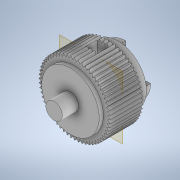
# Autodesk Inventor part: PotAttachmentB10L
Saved by Autodesk Inventor 2022 (Build 260153000, 153)
## iProperties
Created: 2021-10-23
Part Number: PotAttachmentB10L
Material: Generic
Document SubType Name: Modeling
Designer: teh18
Density: 1 g/cm^3
Appearance: Default
Author: teh18
Autodesk Inventor part; units mm, degrees
ref_plane "YZ Plane" through (0, 0, 0) normal (1, 0, 0) x (0, 1, 0)
ref_plane "XZ Plane" through (0, 0, 0) normal (0, 1, 0) x (-1, 0, 0)
ref_plane "XY Plane" through (0, 0, 0) normal (0, 0, 1) x (1, 0, 0)
sketch "Sketch1" plane through (0, 0, 0) normal (0, 0, 1) x (1, 0, 0)
  arc A0 (-0.1225, 6.9989) -> (-6, 3.6056) centre (0, 0) ccw projected
  circle A1 centre (0, 0) radius 7
  line L0 (0, -12) -> (0, -10) projected
  arc A2 (0, -10) -> (10, 0) centre (0, 0) ccw projected
  line L1 (10, 0) -> (12, 0) projected
  arc A3 (0, -12) -> (12, 0) centre (0, 0) ccw projected
  line L2 (0, 12) -> (0, 10) projected
  arc A4 (0, 10) -> (-10, 0) centre (0, 0) ccw projected
  line L3 (-10, 0) -> (-12, 0) projected
  arc A5 (0, 12) -> (-12, 0) centre (0, 0) ccw projected
  arc A6 (4.4269, -19.95) -> (6.1412, -19.4907) centre (5.1647, -19.275) ccw projected
  arc A7 (13.8088, -15.0638) -> (6.1412, -19.4907) centre (12, -20.7846) ccw projected
  arc A8 (13.8088, -15.0638) -> (15.0638, -13.8088) centre (14.1103, -14.1103) ccw projected
  arc A9 (19.4907, -6.1412) -> (15.0638, -13.8088) centre (20.7846, -12) ccw projected
  arc A10 (19.4907, -6.1412) -> (19.95, -4.4269) centre (19.275, -5.1647) ccw projected
  arc A11 (27.8571, 4.5959) -> (19.95, -4.4269) centre (24, 0) ccw projected
  arc A12 (27.8571, 4.5959) -> (29.4828, 5.5468) centre (28.5, 5.3619) ccw projected
  arc A13 (29.4828, 5.5468) -> (27.5804, 11.8035) centre (0, 0) ccw projected
  line L4 (27.5804, 11.8035) -> (33.0964, 14.1643) projected
  arc A14 (33.0964, 14.1643) -> (26.445, 24.4267) centre (0, 0) ccw projected
  line L5 (26.445, 24.4267) -> (22.0375, 20.3556) projected
  arc A15 (22.0375, 20.3556) -> (-20.3556, 22.0375) centre (0, 0) ccw projected
  line L6 (-20.3556, 22.0375) -> (-16.2845, 17.63) projected
  arc A16 (-16.2845, 17.63) -> (-5.9529, -23.25) centre (0, 0) ccw projected
  arc A17 (4.4269, -19.95) -> (-5.9529, -23.25) centre (0, -24) ccw projected
  arc A18 (-1, 6.9282) -> (-6.9282, 1) centre (0, 0) ccw projected
  line L7 (-1, 6.9282) -> (-1, 1) projected
  line L8 (-1, 1) -> (-6.9282, 1) projected
  line L9 (-6.9282, -1) -> (-1, -1) projected
  line L10 (-1, -1) -> (-1, -6.9282) projected
  arc A19 (-6.9282, -1) -> (-1, -6.9282) centre (0, 0) ccw projected
  line L11 (1, -6.9282) -> (1, -1) projected
  line L12 (1, -1) -> (6.9282, -1) projected
  arc A20 (1, -6.9282) -> (6.9282, -1) centre (0, 0) ccw projected
  line L13 (6.9282, 1) -> (1, 1) projected
  line L14 (1, 1) -> (1, 6.9282) projected
  arc A21 (6.9282, 1) -> (1, 6.9282) centre (0, 0) ccw projected
  circle A22 centre (0, 0) radius 14
  point P0 (0, 0)
  point P1 (-6, 3.6056)
  point P2 (-0.1225, 6.9989)
  dimension "d2" = 28
  constraints: 1 centre point, 1 coincident, 2 other
  measures "d2" diameter of A22
extrude "Extrusion1" add sketch "Sketch1" along normal blind 23 contours L0 A2 L1 A3 | L2 A4 L3 A5 | A22
sketch "Sketch2" plane through (0, 0, 0) normal (0, 0, -1) x (-1, 0, 0)
  line L0 (0, -12) -> (0, -10) projected
  arc A0 (-10, 0) -> (0, -10) centre (0, 0) ccw projected
  line L1 (-10, 0) -> (-12, 0) projected
  arc A1 (-12, 0) -> (0, -12) centre (0, 0) ccw projected
  line L2 (0, 12) -> (0, 10) projected
  arc A2 (10, 0) -> (0, 10) centre (0, 0) ccw projected
  line L3 (10, 0) -> (12, 0) projected
  arc A3 (12, 0) -> (0, 12) centre (0, 0) ccw projected
  arc A4 (-6.1412, -19.4907) -> (-4.4269, -19.95) centre (-5.1647, -19.275) ccw projected
  arc A5 (-6.1412, -19.4907) -> (-13.8088, -15.0638) centre (-12, -20.7846) ccw projected
  arc A6 (-15.0638, -13.8088) -> (-13.8088, -15.0638) centre (-14.1103, -14.1103) ccw projected
  arc A7 (-15.0638, -13.8088) -> (-19.4907, -6.1412) centre (-20.7846, -12) ccw projected
  arc A8 (-19.95, -4.4269) -> (-19.4907, -6.1412) centre (-19.275, -5.1647) ccw projected
  arc A9 (-19.95, -4.4269) -> (-27.8571, 4.5959) centre (-24, 0) ccw projected
  arc A10 (-29.4828, 5.5468) -> (-27.8571, 4.5959) centre (-28.5, 5.3619) ccw projected
  arc A11 (-27.5804, 11.8035) -> (-29.4828, 5.5468) centre (0, 0) ccw projected
  line L4 (-27.5804, 11.8035) -> (-33.0964, 14.1643) projected
  arc A12 (-26.445, 24.4267) -> (-33.0964, 14.1643) centre (0, 0) ccw projected
  line L5 (-26.445, 24.4267) -> (-22.0375, 20.3556) projected
  arc A13 (20.3556, 22.0375) -> (-22.0375, 20.3556) centre (0, 0) ccw projected
  line L6 (20.3556, 22.0375) -> (16.2845, 17.63) projected
  arc A14 (5.9529, -23.25) -> (16.2845, 17.63) centre (0, 0) ccw projected
  arc A15 (5.9529, -23.25) -> (-4.4269, -19.95) centre (0, -24) ccw projected
  arc A16 (6.9282, 1) -> (1, 6.9282) centre (0, 0) ccw projected
  line L7 (1, 6.9282) -> (1, 1) projected
  line L8 (1, 1) -> (6.9282, 1) projected
  line L9 (6.9282, -1) -> (1, -1) projected
  line L10 (1, -1) -> (1, -6.9282) projected
  arc A17 (1, -6.9282) -> (6.9282, -1) centre (0, 0) ccw projected
  line L11 (-1, -6.9282) -> (-1, -1) projected
  line L12 (-1, -1) -> (-6.9282, -1) projected
  arc A18 (-6.9282, -1) -> (-1, -6.9282) centre (0, 0) ccw projected
  line L13 (-6.9282, 1) -> (-1, 1) projected
  line L14 (-1, 1) -> (-1, 6.9282) projected
  arc A19 (-1, 6.9282) -> (-6.9282, 1) centre (0, 0) ccw projected
  point P0 (0, 0)
extrude "Extrusion2" add sketch "Sketch2" along normal blind 4 contours A1 L1 A0 L0 | A3 L3 A2 L2
ref_plane "Work Plane1" through (0, 0, 13) normal (0, 0, 1) x (1, 0, 0)
sketch "Sketch4" plane through (0, 0, 13) normal (0, 0, 1) x (1, 0, 0)
  circle A0 centre (0, 0) radius 3
  circle A1 centre (0, 0) radius 7 projected
  dimension "d10" = 6
  constraints: 1 centre point, 1 coincident
  measures "d10" diameter of A0
extrude "Extrusion4" add sketch "Sketch4" along normal up to surface (10 mm away) contours A0 | A1
sketch "Sketch6" plane through (0, 0, 23) normal (0, 0, 1) x (1, 0, 0)
  circle A0 centre (0, 0) radius 4
  dimension "d25" = 8
  constraints: 1 centre point, 1 coincident
  measures "d25" diameter of A0
extrude "Extrusion6" add sketch "Sketch6" along normal blind 8
sketch "Sketch7" plane through (0, 0, 13) normal (0, 0, 1) x (1, 0, 0)
  circle A0 centre (0, 0) radius 14 projected
  line L0 (0, 17.4641) -> (3, 12.2679)
  line L1 (3, 12.2679) -> (-3, 12.2679)
  line L2 (-3, 12.2679) -> (0, 17.4641)
  line L3 (-1.8255, 17.3684) -> (1.7012, 12.5143)
  line L4 (-4.2659, 11.8872) -> (-1.8255, 17.3684)
  line L5 (1.7012, 12.5143) -> (-4.2659, 11.8872)
  line L6 (-3.631, 17.0825) -> (0.3838, 12.6236)
  line L7 (-5.4851, 11.3761) -> (-3.631, 17.0825)
  line L8 (0.3838, 12.6236) -> (-5.4851, 11.3761)
  line L9 (-5.3967, 16.6093) -> (-0.9378, 12.5946)
  line L10 (-6.6442, 10.7405) -> (-5.3967, 16.6093)
  line L11 (-0.9378, 12.5946) -> (-6.6442, 10.7405)
  line L12 (-7.1033, 15.9543) -> (-2.2492, 12.4275)
  line L13 (-7.7305, 9.9871) -> (-7.1033, 15.9543)
  line L14 (-2.2492, 12.4275) -> (-7.7305, 9.9871)
  line L15 (-8.7321, 15.1244) -> (-3.5359, 12.1244)
  line L16 (-8.7321, 9.1244) -> (-8.7321, 15.1244)
  line L17 (-3.5359, 12.1244) -> (-8.7321, 9.1244)
  line L18 (-10.2651, 14.1288) -> (-4.7839, 11.6883)
  line L19 (-9.638, 8.1616) -> (-10.2651, 14.1288)
  line L20 (-4.7839, 11.6883) -> (-9.638, 8.1616)
  line L21 (-11.6858, 12.9784) -> (-5.9794, 11.1243)
  line L22 (-10.4383, 7.1095) -> (-11.6858, 12.9784)
  line L23 (-5.9794, 11.1243) -> (-10.4383, 7.1095)
  line L24 (-12.9784, 11.6858) -> (-7.1095, 10.4383)
  line L25 (-11.1243, 5.9794) -> (-12.9784, 11.6858)
  line L26 (-7.1095, 10.4383) -> (-11.1243, 5.9794)
  line L27 (-14.1288, 10.2651) -> (-8.1616, 9.638)
  line L28 (-11.6883, 4.7839) -> (-14.1288, 10.2651)
  line L29 (-8.1616, 9.638) -> (-11.6883, 4.7839)
  line L30 (-15.1244, 8.7321) -> (-9.1244, 8.7321)
  line L31 (-12.1244, 3.5359) -> (-15.1244, 8.7321)
  line L32 (-9.1244, 8.7321) -> (-12.1244, 3.5359)
  line L33 (-15.9543, 7.1033) -> (-9.9871, 7.7305)
  line L34 (-12.4275, 2.2492) -> (-15.9543, 7.1033)
  line L35 (-9.9871, 7.7305) -> (-12.4275, 2.2492)
  line L36 (-16.6093, 5.3967) -> (-10.7405, 6.6442)
  line L37 (-12.5946, 0.9378) -> (-16.6093, 5.3967)
  line L38 (-10.7405, 6.6442) -> (-12.5946, 0.9378)
  line L39 (-17.0825, 3.631) -> (-11.3761, 5.4851)
  line L40 (-12.6236, -0.3838) -> (-17.0825, 3.631)
  line L41 (-11.3761, 5.4851) -> (-12.6236, -0.3838)
  line L42 (-17.3684, 1.8255) -> (-11.8872, 4.2659)
  line L43 (-12.5143, -1.7012) -> (-17.3684, 1.8255)
  line L44 (-11.8872, 4.2659) -> (-12.5143, -1.7012)
  line L45 (-17.4641, 0) -> (-12.2679, 3)
  line L46 (-12.2679, -3) -> (-17.4641, 0)
  line L47 (-12.2679, 3) -> (-12.2679, -3)
  line L48 (-17.3684, -1.8255) -> (-12.5143, 1.7012)
  line L49 (-11.8872, -4.2659) -> (-17.3684, -1.8255)
  line L50 (-12.5143, 1.7012) -> (-11.8872, -4.2659)
  line L51 (-17.0825, -3.631) -> (-12.6236, 0.3838)
  line L52 (-11.3761, -5.4851) -> (-17.0825, -3.631)
  line L53 (-12.6236, 0.3838) -> (-11.3761, -5.4851)
  line L54 (-16.6093, -5.3967) -> (-12.5946, -0.9378)
  line L55 (-10.7405, -6.6442) -> (-16.6093, -5.3967)
  line L56 (-12.5946, -0.9378) -> (-10.7405, -6.6442)
  line L57 (-15.9543, -7.1033) -> (-12.4275, -2.2492)
  line L58 (-9.9871, -7.7305) -> (-15.9543, -7.1033)
  line L59 (-12.4275, -2.2492) -> (-9.9871, -7.7305)
  line L60 (-15.1244, -8.7321) -> (-12.1244, -3.5359)
  line L61 (-9.1244, -8.7321) -> (-15.1244, -8.7321)
  line L62 (-12.1244, -3.5359) -> (-9.1244, -8.7321)
  line L63 (-14.1288, -10.2651) -> (-11.6883, -4.7839)
  line L64 (-8.1616, -9.638) -> (-14.1288, -10.2651)
  line L65 (-11.6883, -4.7839) -> (-8.1616, -9.638)
  line L66 (-12.9784, -11.6858) -> (-11.1243, -5.9794)
  line L67 (-7.1095, -10.4383) -> (-12.9784, -11.6858)
  line L68 (-11.1243, -5.9794) -> (-7.1095, -10.4383)
  line L69 (-11.6858, -12.9784) -> (-10.4383, -7.1095)
  line L70 (-5.9794, -11.1243) -> (-11.6858, -12.9784)
  line L71 (-10.4383, -7.1095) -> (-5.9794, -11.1243)
  line L72 (-10.2651, -14.1288) -> (-9.638, -8.1616)
  line L73 (-4.7839, -11.6883) -> (-10.2651, -14.1288)
  line L74 (-9.638, -8.1616) -> (-4.7839, -11.6883)
  line L75 (-8.7321, -15.1244) -> (-8.7321, -9.1244)
  line L76 (-3.5359, -12.1244) -> (-8.7321, -15.1244)
  line L77 (-8.7321, -9.1244) -> (-3.5359, -12.1244)
  line L78 (-7.1033, -15.9543) -> (-7.7305, -9.9871)
  line L79 (-2.2492, -12.4275) -> (-7.1033, -15.9543)
  line L80 (-7.7305, -9.9871) -> (-2.2492, -12.4275)
  line L81 (-5.3967, -16.6093) -> (-6.6442, -10.7405)
  line L82 (-0.9378, -12.5946) -> (-5.3967, -16.6093)
  line L83 (-6.6442, -10.7405) -> (-0.9378, -12.5946)
  line L84 (-3.631, -17.0825) -> (-5.4851, -11.3761)
  line L85 (0.3838, -12.6236) -> (-3.631, -17.0825)
  line L86 (-5.4851, -11.3761) -> (0.3838, -12.6236)
  line L87 (-1.8255, -17.3684) -> (-4.2659, -11.8872)
  line L88 (1.7012, -12.5143) -> (-1.8255, -17.3684)
  line L89 (-4.2659, -11.8872) -> (1.7012, -12.5143)
  line L90 (0, -17.4641) -> (-3, -12.2679)
  line L91 (3, -12.2679) -> (0, -17.4641)
  line L92 (-3, -12.2679) -> (3, -12.2679)
  line L93 (1.8255, -17.3684) -> (-1.7012, -12.5143)
  line L94 (4.2659, -11.8872) -> (1.8255, -17.3684)
  line L95 (-1.7012, -12.5143) -> (4.2659, -11.8872)
  line L96 (3.631, -17.0825) -> (-0.3838, -12.6236)
  line L97 (5.4851, -11.3761) -> (3.631, -17.0825)
  line L98 (-0.3838, -12.6236) -> (5.4851, -11.3761)
  line L99 (5.3967, -16.6093) -> (0.9378, -12.5946)
  line L100 (6.6442, -10.7405) -> (5.3967, -16.6093)
  line L101 (0.9378, -12.5946) -> (6.6442, -10.7405)
  line L102 (7.1033, -15.9543) -> (2.2492, -12.4275)
  line L103 (7.7305, -9.9871) -> (7.1033, -15.9543)
  line L104 (2.2492, -12.4275) -> (7.7305, -9.9871)
  line L105 (8.7321, -15.1244) -> (3.5359, -12.1244)
  line L106 (8.7321, -9.1244) -> (8.7321, -15.1244)
  line L107 (3.5359, -12.1244) -> (8.7321, -9.1244)
  line L108 (10.2651, -14.1288) -> (4.7839, -11.6883)
  line L109 (9.638, -8.1616) -> (10.2651, -14.1288)
  line L110 (4.7839, -11.6883) -> (9.638, -8.1616)
  line L111 (11.6858, -12.9784) -> (5.9794, -11.1243)
  line L112 (10.4383, -7.1095) -> (11.6858, -12.9784)
  line L113 (5.9794, -11.1243) -> (10.4383, -7.1095)
  line L114 (12.9784, -11.6858) -> (7.1095, -10.4383)
  line L115 (11.1243, -5.9794) -> (12.9784, -11.6858)
  line L116 (7.1095, -10.4383) -> (11.1243, -5.9794)
  line L117 (14.1288, -10.2651) -> (8.1616, -9.638)
  line L118 (11.6883, -4.7839) -> (14.1288, -10.2651)
  line L119 (8.1616, -9.638) -> (11.6883, -4.7839)
  line L120 (15.1244, -8.7321) -> (9.1244, -8.7321)
  line L121 (12.1244, -3.5359) -> (15.1244, -8.7321)
  line L122 (9.1244, -8.7321) -> (12.1244, -3.5359)
  line L123 (15.9543, -7.1033) -> (9.9871, -7.7305)
  line L124 (12.4275, -2.2492) -> (15.9543, -7.1033)
  line L125 (9.9871, -7.7305) -> (12.4275, -2.2492)
  line L126 (16.6093, -5.3967) -> (10.7405, -6.6442)
  line L127 (12.5946, -0.9378) -> (16.6093, -5.3967)
  line L128 (10.7405, -6.6442) -> (12.5946, -0.9378)
  line L129 (17.0825, -3.631) -> (11.3761, -5.4851)
  line L130 (12.6236, 0.3838) -> (17.0825, -3.631)
  line L131 (11.3761, -5.4851) -> (12.6236, 0.3838)
  line L132 (17.3684, -1.8255) -> (11.8872, -4.2659)
  line L133 (12.5143, 1.7012) -> (17.3684, -1.8255)
  line L134 (11.8872, -4.2659) -> (12.5143, 1.7012)
  line L135 (17.4641, 0) -> (12.2679, -3)
  line L136 (12.2679, 3) -> (17.4641, 0)
  line L137 (12.2679, -3) -> (12.2679, 3)
  line L138 (17.3684, 1.8255) -> (12.5143, -1.7012)
  line L139 (11.8872, 4.2659) -> (17.3684, 1.8255)
  line L140 (12.5143, -1.7012) -> (11.8872, 4.2659)
  line L141 (17.0825, 3.631) -> (12.6236, -0.3838)
  line L142 (11.3761, 5.4851) -> (17.0825, 3.631)
  line L143 (12.6236, -0.3838) -> (11.3761, 5.4851)
  line L144 (16.6093, 5.3967) -> (12.5946, 0.9378)
  line L145 (10.7405, 6.6442) -> (16.6093, 5.3967)
  line L146 (12.5946, 0.9378) -> (10.7405, 6.6442)
  line L147 (15.9543, 7.1033) -> (12.4275, 2.2492)
  line L148 (9.9871, 7.7305) -> (15.9543, 7.1033)
  line L149 (12.4275, 2.2492) -> (9.9871, 7.7305)
  line L150 (15.1244, 8.7321) -> (12.1244, 3.5359)
  line L151 (9.1244, 8.7321) -> (15.1244, 8.7321)
  line L152 (12.1244, 3.5359) -> (9.1244, 8.7321)
  line L153 (14.1288, 10.2651) -> (11.6883, 4.7839)
  line L154 (8.1616, 9.638) -> (14.1288, 10.2651)
  line L155 (11.6883, 4.7839) -> (8.1616, 9.638)
  line L156 (12.9784, 11.6858) -> (11.1243, 5.9794)
  line L157 (7.1095, 10.4383) -> (12.9784, 11.6858)
  line L158 (11.1243, 5.9794) -> (7.1095, 10.4383)
  line L159 (11.6858, 12.9784) -> (10.4383, 7.1095)
  line L160 (5.9794, 11.1243) -> (11.6858, 12.9784)
  line L161 (10.4383, 7.1095) -> (5.9794, 11.1243)
  line L162 (10.2651, 14.1288) -> (9.638, 8.1616)
  line L163 (4.7839, 11.6883) -> (10.2651, 14.1288)
  line L164 (9.638, 8.1616) -> (4.7839, 11.6883)
  line L165 (8.7321, 15.1244) -> (8.7321, 9.1244)
  line L166 (3.5359, 12.1244) -> (8.7321, 15.1244)
  line L167 (8.7321, 9.1244) -> (3.5359, 12.1244)
  line L168 (7.1033, 15.9543) -> (7.7305, 9.9871)
  line L169 (2.2492, 12.4275) -> (7.1033, 15.9543)
  line L170 (7.7305, 9.9871) -> (2.2492, 12.4275)
  line L171 (5.3967, 16.6093) -> (6.6442, 10.7405)
  line L172 (0.9378, 12.5946) -> (5.3967, 16.6093)
  line L173 (6.6442, 10.7405) -> (0.9378, 12.5946)
  line L174 (3.631, 17.0825) -> (5.4851, 11.3761)
  line L175 (-0.3838, 12.6236) -> (3.631, 17.0825)
  line L176 (5.4851, 11.3761) -> (-0.3838, 12.6236)
  line L177 (1.8255, 17.3684) -> (4.2659, 11.8872)
  line L178 (-1.7012, 12.5143) -> (1.8255, 17.3684)
  line L179 (4.2659, 11.8872) -> (-1.7012, 12.5143)
  point P0 (0, 0)
  point P1 (0, 14)
  point P2 (-1.4634, 13.9233)
  point P3 (-2.9108, 13.6941)
  point P4 (-4.3262, 13.3148)
  point P5 (-5.6943, 12.7896)
  point P6 (-7, 12.1244)
  point P7 (-8.229, 11.3262)
  point P8 (-9.3678, 10.404)
  point P9 (-10.404, 9.3678)
  point P10 (-11.3262, 8.229)
  point P11 (-12.1244, 7)
  point P12 (-12.7896, 5.6943)
  point P13 (-13.3148, 4.3262)
  point P14 (-13.6941, 2.9108)
  point P15 (-13.9233, 1.4634)
  point P16 (-14, 0)
  point P17 (-13.9233, -1.4634)
  point P18 (-13.6941, -2.9108)
  point P19 (-13.3148, -4.3262)
  point P20 (-12.7896, -5.6943)
  point P21 (-12.1244, -7)
  point P22 (-11.3262, -8.229)
  point P23 (-10.404, -9.3678)
  point P24 (-9.3678, -10.404)
  point P25 (-8.229, -11.3262)
  point P26 (-7, -12.1244)
  point P27 (-5.6943, -12.7896)
  point P28 (-4.3262, -13.3148)
  point P29 (-2.9108, -13.6941)
  point P30 (-1.4634, -13.9233)
  point P31 (0, -14)
  point P32 (1.4634, -13.9233)
  point P33 (2.9108, -13.6941)
  point P34 (4.3262, -13.3148)
  point P35 (5.6943, -12.7896)
  point P36 (7, -12.1244)
  point P37 (8.229, -11.3262)
  point P38 (9.3678, -10.404)
  point P39 (10.404, -9.3678)
  point P40 (11.3262, -8.229)
  point P41 (12.1244, -7)
  point P42 (12.7896, -5.6943)
  point P43 (13.3148, -4.3262)
  point P44 (13.6941, -2.9108)
  point P45 (13.9233, -1.4634)
  point P46 (14, 0)
  point P47 (13.9233, 1.4634)
  point P48 (13.6941, 2.9108)
  point P49 (13.3148, 4.3262)
  point P50 (12.7896, 5.6943)
  point P51 (12.1244, 7)
  point P52 (11.3262, 8.229)
  point P53 (10.404, 9.3678)
  point P54 (9.3678, 10.404)
  point P55 (8.229, 11.3262)
  point P56 (7, 12.1244)
  point P57 (5.6943, 12.7896)
  point P58 (4.3262, 13.3148)
  point P59 (2.9108, 13.6941)
  point P60 (1.4634, 13.9233)
  point P61 (0.8332, 13.9752)
  point P62 (3.5262, 13.5487)
  point P63 (-0.6322, 13.9857)
  point P64 (2.0906, 13.843)
  point P65 (-2.0906, 13.843)
  point P66 (0.6322, 13.9857)
  point P67 (-3.5262, 13.5487)
  point P68 (-0.8332, 13.9752)
  point P69 (-4.9231, 13.1059)
  point P70 (-2.2894, 13.8115)
  point P71 (-6.266, 12.5195)
  point P72 (-3.7206, 13.4966)
  point P73 (-7.5404, 11.7959)
  point P74 (-5.111, 13.0337)
  point P75 (-8.7321, 10.9431)
  point P76 (-6.4454, 12.4281)
  point P77 (-9.8281, 9.9704)
  point P78 (-7.7091, 11.6863)
  point P79 (-10.8164, 8.8885)
  point P80 (-8.8885, 10.8164)
  point P81 (-11.6863, 7.7091)
  point P82 (-9.9704, 9.8281)
  point P83 (-12.4281, 6.4454)
  point P84 (-10.9431, 8.7321)
  point P85 (-13.0337, 5.111)
  point P86 (-11.7959, 7.5404)
  point P87 (-13.4966, 3.7206)
  point P88 (-12.5195, 6.266)
  point P89 (-13.8115, 2.2894)
  point P90 (-13.1059, 4.9231)
  point P91 (-13.9752, 0.8332)
  point P92 (-13.5487, 3.5262)
  point P93 (-13.9857, -0.6322)
  point P94 (-13.843, 2.0906)
  point P95 (-13.843, -2.0906)
  point P96 (-13.9857, 0.6322)
  point P97 (-13.5487, -3.5262)
  point P98 (-13.9752, -0.8332)
  point P99 (-13.1059, -4.9231)
  point P100 (-13.8115, -2.2894)
  point P101 (-12.5195, -6.266)
  point P102 (-13.4966, -3.7206)
  point P103 (-11.7959, -7.5404)
  point P104 (-13.0337, -5.111)
  point P105 (-10.9431, -8.7321)
  point P106 (-12.4281, -6.4454)
  point P107 (-9.9704, -9.8281)
  point P108 (-11.6863, -7.7091)
  point P109 (-8.8885, -10.8164)
  point P110 (-10.8164, -8.8885)
  point P111 (-7.7091, -11.6863)
  point P112 (-9.8281, -9.9704)
  point P113 (-6.4454, -12.4281)
  point P114 (-8.7321, -10.9431)
  point P115 (-5.111, -13.0337)
  point P116 (-7.5404, -11.7959)
  point P117 (-3.7206, -13.4966)
  point P118 (-6.266, -12.5195)
  point P119 (-2.2894, -13.8115)
  point P120 (-4.9231, -13.1059)
  point P121 (-0.8332, -13.9752)
  point P122 (-3.5262, -13.5487)
  point P123 (0.6322, -13.9857)
  point P124 (-2.0906, -13.843)
  point P125 (2.0906, -13.843)
  point P126 (-0.6322, -13.9857)
  point P127 (3.5262, -13.5487)
  point P128 (0.8332, -13.9752)
  point P129 (4.9231, -13.1059)
  point P130 (2.2894, -13.8115)
  point P131 (6.266, -12.5195)
  point P132 (3.7206, -13.4966)
  point P133 (7.5404, -11.7959)
  point P134 (5.111, -13.0337)
  point P135 (8.7321, -10.9431)
  point P136 (6.4454, -12.4281)
  point P137 (9.8281, -9.9704)
  point P138 (7.7091, -11.6863)
  point P139 (10.8164, -8.8885)
  point P140 (8.8885, -10.8164)
  point P141 (11.6863, -7.7091)
  point P142 (9.9704, -9.8281)
  point P143 (12.4281, -6.4454)
  point P144 (10.9431, -8.7321)
  point P145 (13.0337, -5.111)
  point P146 (11.7959, -7.5404)
  point P147 (13.4966, -3.7206)
  point P148 (12.5195, -6.266)
  point P149 (13.8115, -2.2894)
  point P150 (13.1059, -4.9231)
  point P151 (13.9752, -0.8332)
  point P152 (13.5487, -3.5262)
  point P153 (13.9857, 0.6322)
  point P154 (13.843, -2.0906)
  point P155 (13.843, 2.0906)
  point P156 (13.9857, -0.6322)
  point P157 (13.5487, 3.5262)
  point P158 (13.9752, 0.8332)
  point P159 (13.1059, 4.9231)
  point P160 (13.8115, 2.2894)
  point P161 (12.5195, 6.266)
  point P162 (13.4966, 3.7206)
  point P163 (11.7959, 7.5404)
  point P164 (13.0337, 5.111)
  point P165 (10.9431, 8.7321)
  point P166 (12.4281, 6.4454)
  point P167 (9.9704, 9.8281)
  point P168 (11.6863, 7.7091)
  point P169 (8.8885, 10.8164)
  point P170 (10.8164, 8.8885)
  point P171 (7.7091, 11.6863)
  point P172 (9.8281, 9.9704)
  point P173 (6.4454, 12.4281)
  point P174 (8.7321, 10.9431)
  point P175 (5.111, 13.0337)
  point P176 (7.5404, 11.7959)
  point P177 (3.7206, 13.4966)
  point P178 (6.266, 12.5195)
  point P179 (2.2894, 13.8115)
  point P180 (4.9231, 13.1059)
  point P181 (-0.6429, 12.2679)
  point P182 (0.6429, 12.2679)
  point P183 (1.9218, 12.1335)
  point P184 (3.1795, 11.8662)
  point P185 (4.4025, 11.4688)
  point P186 (5.5772, 10.9458)
  point P187 (6.6908, 10.3029)
  point P188 (7.7311, 9.5471)
  point P189 (8.6867, 8.6867)
  point P190 (9.5471, 7.7311)
  point P191 (10.3029, 6.6908)
  point P192 (10.9458, 5.5772)
  point P193 (11.4688, 4.4025)
  point P194 (11.8662, 3.1795)
  point P195 (12.1335, 1.9218)
  point P196 (12.2679, 0.6429)
  point P197 (12.2679, -0.6429)
  point P198 (12.1335, -1.9218)
  point P199 (11.8662, -3.1795)
  dimension "d28" = 6
  dimension "d31" = 360
  constraints: 360 end point, 1 horizontal alignment, 1 vertical alignment, 429 other
  measures "d28" distance of L0.end L1.end
extrude "Extrusion7" add sketch "Sketch7" along normal mid plane 16 contours A0 L138 L130 L141 L133 | A0 L133 L138 | L133 L141 A0 | A0 L141 L136 L138 L133 | L138 L133 L135 L130 A0 | A0 L130 L138 | L141 L133 L144 L136 A0 | A0 L136 L141 | L141 L130 L131 L143 L134 L146 L144 L133 | L138 L136 L135 L133 | L130 L135 A0 | A0 L135 L127 L138 L130 | L138 L127 L128 L140 L131 L143 L141 L130 | L136 L144 A0 | A0 L144 L139 L141 L136 | L141 L139 L138 L136 | L144 L146 L134 L133 | L133 L134 L146 L137 L149 L147 L136 L144 | L141 L143 L131 L130 | L133 L132 L130 L135 | L135 L130 L132 L127 A0 | A0 L127 L135 | L138 L140 L128 L127 | L127 L135 L124 L125 L137 L128 L140 L138 | L144 L136 L147 L139 A0 | A0 L139 L144 | L139 L144 L142 L141 | L127 L132 A0 | A0 L132 L124 L135 L127 | L130 L129 L127 L132 | L139 L147 A0 | A0 L147 L142 L144 L139 | L136 L137 L149 L140 L152 L150 L139 L147 | L134 L143 L137 L146 | L131 L140 L134 L143 | L132 L127 L129 L124 A0 | A0 L124 L132 | L135 L137 L125 L124 | L124 L132 L121 L122 L134 L125 L137 L135 | L128 L137 L131 L140 | L147 L139 L150 L142 A0 | A0 L142 L147 | L142 L147 L145 L144 | L134 L140 L137 L143 | L146 L140 L149 L137 | L137 L143 L140 L146 | L131 L137 L134 L140 | L124 L129 A0 | A0 L129 L121 L132 L124 | L127 L126 L124 L129 | L137 L125 L134 L128 | L128 L134 L131 L137 | L142 L150 A0 | A0 L150 L145 L147 L142 | L150 L152 L140 L139 | L139 L140 L152 L143 L155 L153 L142 L150 | L134 L137 L140 | L137 L140 L143 | L146 L143 L149 L140 | L140 L143 L146 | L131 L134 L137 | L129 L124 L126 L121 A0 | A0 L121 L129 | L132 L134 L122 L121 | L121 L129 L118 L119 L131 L122 L134 L132 | L134 L125 L131 L128 | L128 L131 L134 | L150 L142 L153 L145 A0 | A0 L145 L150 | L145 L150 L148 L147 | L149 L143 L152 L140 | L146 L149 L143 | L121 L126 A0 | A0 L126 L118 L129 L121 | L124 L123 L121 L126 | L134 L122 L131 L125 | L131 L125 L128 | L145 L153 A0 | A0 L153 L148 L150 L145 | L153 L155 L143 L142 | L142 L143 L155 L146 L158 L156 L145 L153 | L149 L146 L152 L143 | L149 L152 L146 | L126 L121 L123 L118 A0 | A0 L118 L126 | L129 L131 L119 L118 | L118 L126 L115 L116 L128 L119 L131 L129 | L131 L122 L128 L125 | L128 L122 L125 | L153 L145 L156 L148 A0 | A0 L148 L153 | L148 L153 L151 L150 | L152 L146 L155 L143 | L152 L149 L155 L146 | L152 L155 L149 | L118 L123 A0 | A0 L123 L115 L126 L118 | L121 L120 L118 L123 | L131 L119 L128 L122 | L125 L119 L122 | L122 L128 L119 L125 | L148 L156 A0 | A0 L156 L151 L153 L148 | L156 L158 L146 L145 | L145 L146 L158 L149 L161 L159 L148 L156 | L155 L149 L158 L146 | L155 L152 L158 L149 | L155 L158 L152 | L123 L118 L120 L115 A0 | A0 L115 L123 | L126 L128 L116 L115 | L115 L123 L112 L113 L125 L116 L128 L126 | L122 L116 L119 | L119 L125 L116 L122 | L119 L128 L116 L125 | L156 L148 L159 L151 A0 | A0 L151 L156 | L151 L156 L154 L153 | L158 L152 L161 L149 | L158 L155 L161 L152 | L158 L161 L155 | L115 L120 A0 | A0 L120 L112 L123 L115 | L118 L117 L115 L120 | L119 L113 L116 | L116 L122 L113 L119 | L116 L125 L113 L122 | L151 L159 A0 | A0 L159 L154 L156 L151 | L159 L161 L149 L148 | L148 L149 L161 L152 L164 L162 L151 L159 | L161 L155 L164 L152 | L161 L158 L164 L155 | L161 L164 L158 | L120 L115 L117 L112 A0 | A0 L112 L120 | L123 L125 L113 L112 | L112 L120 L109 L110 L122 L113 L125 L123 | L116 L110 L113 | L113 L119 L110 L116 | L113 L122 L110 L119 | L159 L151 L162 L154 A0 | A0 L154 L159 | L154 L159 L157 L156 | L164 L155 L167 L165 L154 L162 L151 L152 | L152 L151 L162 L164 | L164 L158 L167 L155 | L164 L161 L167 L158 | L164 L167 L161 | L112 L117 A0 | A0 L117 L109 L120 L112 | L115 L114 L112 L117 | L113 L107 L110 | L110 L116 L107 L113 | L110 L119 L107 L116 | L110 L122 L120 L109 L117 L106 L107 L119 | L110 L109 L120 L122 | L154 L162 A0 | A0 L162 L157 L159 L154 | L167 L158 L170 L168 L157 L165 L154 L155 | L155 L154 L165 L167 | L167 L161 L170 L158 | L167 L164 L170 L161 | L167 L170 L164 | L117 L112 L114 L109 A0 | A0 L109 L117 | L110 L104 L107 | L107 L113 L104 L110 | L107 L116 L104 L113 | L107 L119 L117 L106 L114 L103 L104 L116 | L107 L106 L117 L119 | L162 L154 L165 L157 A0 | A0 L157 L162 | L157 L162 L160 L159 | L170 L161 L173 L171 L160 L168 L157 L158 | L158 L157 L168 L170 | L170 L164 L173 L161 | L170 L167 L173 L164 | L170 L173 L167 | L109 L114 A0 | A0 L114 L106 L117 L109 | L112 L111 L109 L114 | L107 L101 L104 | L104 L110 L101 L107 | L104 L113 L101 L110 | L104 L116 L114 L103 L111 L100 L101 L113 | L104 L103 L114 L116 | L157 L165 A0 | A0 L165 L160 L162 L157 | L173 L164 L176 L174 L163 L171 L160 L161 | L161 L160 L171 L173 | L173 L167 L176 L164 | L173 L170 L176 L167 | L173 L176 L170 | L114 L109 L111 L106 A0 | A0 L106 L114 | L104 L98 L101 | L101 L107 L98 L104 | L101 L110 L98 L107 | L101 L113 L111 L100 L108 L97 L98 L110 | L101 L100 L111 L113 | L165 L157 L168 L160 A0 | A0 L160 L165 | L160 L165 L163 L162 | L176 L167 L179 L177 L166 L174 L163 L164 | L164 L163 L174 L176 | L176 L170 L179 L167 | L176 L173 L179 L170 | L176 L179 L173 | L106 L111 A0 | A0 L111 L103 L114 L106 | L109 L108 L106 L111 | L101 L95 L98 | L98 L104 L95 L101 | L98 L107 L95 L104 | L98 L110 L108 L97 L105 L94 L95 L107 | L98 L97 L108 L110 | L160 L168 A0 | A0 L168 L163 L165 L160 | L160 L171 L163 A0 L168 | L179 L170 L1 L0 L169 L177 L166 L167 | L167 L166 L177 L179 | L179 L173 L1 L170 | L179 L176 L1 L173 | L179 L1 L176 | L111 L106 L108 L103 A0 | A0 L103 L111 | L98 L92 L95 | L95 L101 L92 L98 | L95 L104 L92 L101 | L95 L107 L105 L94 L102 L91 L92 L104 | L95 L94 L105 L107 | L111 L103 A0 L108 L100 | A0 L163 L168 | L163 L168 L166 L165 | L171 A0 L163 | L163 L174 L166 A0 L171 | L170 L169 L0 L1 | L1 L173 L5 L3 L172 L0 L169 L170 | L1 L176 L5 L173 | L1 L179 L5 L176 | L1 L5 L179 | L103 L108 A0 | L106 L105 L103 L108 | L95 L89 L92 | L92 L98 L89 L95 | L92 L101 L89 L98 | L92 L104 L102 L91 L99 L88 L89 L101 | L92 L91 L102 L104 | L108 L100 A0 L105 L97 | L108 A0 L100 | A0 L171 L166 L168 L163 | A0 L166 L171 | L174 A0 L166 | L166 L177 L169 A0 L174 | L173 L172 L3 L5 | L5 L176 L8 L6 L175 L3 L172 L173 | L5 L179 L8 L176 | L5 L8 L1 | L1 L8 L179 L5 | L108 L103 L105 L100 A0 | L92 L86 L89 | L89 L95 L86 L92 | L89 L98 L86 L95 | L89 L101 L99 L88 L96 L85 L86 L98 | L89 L88 L99 L101 | L105 L97 A0 L102 L94 | L105 A0 L97 | L100 L105 A0 | L166 L171 L169 L168 | A0 L174 L169 L171 L166 | A0 L169 L174 | L177 A0 L169 | L169 L0 L172 A0 L177 | L176 L175 L6 L8 | L8 L179 L11 L9 L178 L6 L175 L176 | L8 L5 L11 L1 | L1 L11 L179 L8 | L8 L11 L5 | L103 L102 L100 L105 | L89 L83 L86 | L86 L92 L83 L89 | L86 L95 L83 L92 | L86 L98 L96 L85 L93 L82 L83 L95 | L86 L85 L96 L98 | L102 L94 A0 L99 L91 | L102 A0 L94 | L97 L102 A0 | A0 L105 L100 L102 L97 | L169 L174 L172 L171 | A0 L177 L172 L174 L169 | A0 L172 L177 | L172 L3 L175 A0 L0 | L0 A0 L172 | L11 L5 L14 L1 | L1 L14 L12 L2 L9 L178 L179 L11 | L11 L8 L14 L5 | L11 L14 L8 | L179 L178 L9 L11 | L86 L80 L83 | L83 L89 L80 L86 | L83 L92 L80 L89 | L83 L95 L93 L82 L90 L79 L80 L92 | L83 L82 L93 L95 | L99 L91 A0 L96 L88 | L99 A0 L91 | L94 L99 A0 | A0 L102 L97 L99 L94 | L102 L100 L99 L97 | L172 L177 L175 L174 | A0 L0 L175 L177 L172 | A0 L175 L0 | L175 L6 L178 A0 L3 | L3 A0 L175 | L14 L5 L17 L15 L4 L12 L2 L1 | L1 L2 L12 L14 | L14 L8 L17 L5 | L14 L11 L17 L8 | L14 L17 L11 | L83 L77 L80 | L80 L86 L77 L83 | L80 L89 L77 L86 | L80 L92 L90 L79 L87 L76 L77 L89 | L80 L79 L90 L92 | L96 L88 A0 L93 L85 | L96 A0 L88 | L91 L96 A0 | A0 L99 L94 L96 L91 | L99 L97 L96 L94 | L175 L0 L178 L177 | A0 L3 L178 L0 L175 | A0 L178 L3 | L178 L9 L2 A0 L6 | L6 A0 L178 | L17 L8 L20 L18 L7 L15 L4 L5 | L5 L4 L15 L17 | L17 L11 L20 L8 | L17 L14 L20 L11 | L17 L20 L14 | L80 L74 L77 | L77 L83 L74 L80 | L77 L86 L74 L83 | L77 L89 L87 L76 L84 L73 L74 L86 | L77 L76 L87 L89 | L93 L85 A0 L90 L82 | L93 A0 L85 | L88 L93 A0 | A0 L96 L91 L93 L88 | L96 L94 L93 L91 | L178 L3 L2 L0 | A0 L6 L2 L3 L178 | A0 L2 L6 | L12 L4 A0 L9 L2 | L20 L11 L23 L21 L10 L18 L7 L8 | L8 L7 L18 L20 | L20 L14 L23 L11 | L20 L17 L23 L14 | L20 L23 L17 | L9 A0 L2 | L77 L71 L74 | L74 L80 L71 L77 | L74 L83 L71 L80 | L74 L86 L84 L73 L81 L70 L71 L83 | L74 L73 L84 L86 | L90 L82 A0 L87 L79 | L90 A0 L82 | L85 L90 A0 | A0 L93 L88 L90 L85 | L93 L91 L90 L88 | L2 L6 L4 L3 | A0 L9 L4 L6 L2 | L12 A0 L4 | L4 L15 L7 A0 L12 | L23 L14 L26 L24 L13 L21 L10 L11 | L11 L10 L21 L23 | L23 L17 L26 L14 | L23 L20 L26 L17 | L23 L26 L20 | A0 L4 L9 | L74 L68 L71 | L71 L77 L68 L74 | L71 L80 L68 L77 | L71 L83 L81 L70 L78 L67 L68 L80 | L71 L70 L81 L83 | L87 L79 A0 L84 L76 | L87 A0 L79 | L82 L87 A0 | A0 L90 L85 L87 L82 | L90 L88 L87 L85 | L4 L9 L7 L6 | A0 L12 L7 L9 L4 | A0 L7 L12 | L15 A0 L7 | L7 L18 L10 A0 L15 | L26 L17 L29 L27 L16 L24 L13 L14 | L14 L13 L24 L26 | L26 L20 L29 L17 | L26 L23 L29 L20 | L26 L29 L23 | L71 L65 L68 | L68 L74 L65 L71 | L68 L77 L65 L74 | L68 L80 L78 L67 L75 L64 L65 L77 | L68 L67 L78 L80 | L84 L76 A0 L81 L73 | L84 A0 L76 | L79 L84 A0 | A0 L87 L82 L84 L79 | L87 L85 L84 L82 | A0 L15 L10 L12 L7 | L12 L10 L9 L7 | A0 L10 L15 | L18 A0 L10 | L10 L21 L13 A0 L18 | L29 L20 L32 L30 L19 L27 L16 L17 | L17 L16 L27 L29 | L29 L23 L32 L20 | L29 L26 L32 L23 | L29 L32 L26 | L68 L62 L65 | L65 L71 L62 L68 | L65 L74 L62 L71 | L65 L77 L75 L64 L72 L61 L62 L74 | L65 L64 L75 L77 | L81 L73 A0 L78 L70 | L81 A0 L73 | L76 L81 A0 | A0 L84 L79 L81 L76 | L84 L82 L81 L79 | L10 L15 L13 L12 | A0 L18 L13 L15 L10 | A0 L13 L18 | L21 A0 L13 | L13 L24 L16 A0 L21 | L32 L23 L35 L33 L22 L30 L19 L20 | L20 L19 L30 L32 | L32 L26 L35 L23 | L32 L29 L35 L26 | L32 L35 L29 | L65 L59 L62 | L62 L68 L59 L65 | L62 L71 L59 L68 | L62 L74 L72 L61 L69 L58 L59 L71 | L62 L61 L72 L74 | L78 L70 A0 L75 L67 | L78 A0 L70 | L73 L78 A0 | A0 L81 L76 L78 L73 | L81 L79 L78 L76 | L13 L18 L16 L15 | A0 L21 L16 L18 L13 | A0 L16 L21 | L24 A0 L16 | L16 L27 L19 A0 L24 | L35 L26 L38 L36 L25 L33 L22 L23 | L23 L22 L33 L35 | L35 L29 L38 L26 | L35 L32 L38 L29 | L35 L38 L32 | L62 L56 L59 | L59 L65 L56 L62 | L59 L68 L56 L65 | L59 L71 L69 L58 L66 L55 L56 L68 | L59 L58 L69 L71 | L75 L67 A0 L72 L64 | L75 A0 L67 | L70 L75 A0 | A0 L78 L73 L75 L70 | L78 L76 L75 L73 | L16 L21 L19 L18 | A0 L24 L19 L21 L16 | A0 L19 L24 | L27 A0 L19 | L19 L30 L22 A0 L27 | L38 L29 L41 L39 L28 L36 L25 L26 | L26 L25 L36 L38 | L38 L32 L41 L29 | L38 L35 L41 L32 | L38 L41 L35 | L59 L53 L56 | L56 L62 L53 L59 | L56 L65 L53 L62 | L56 L68 L66 L55 L63 L52 L53 L65 | L56 L55 L66 L68 | L72 L64 A0 L69 L61 | L72 A0 L64 | L67 L72 A0 | A0 L75 L70 L72 L67 | L75 L73 L72 L70 | L19 L24 L22 L21 | A0 L27 L22 L24 L19 | A0 L22 L27 | L30 A0 L22 | L22 L33 L25 A0 L30 | L41 L32 L44 L42 L31 L39 L28 L29 | L29 L28 L39 L41 | L41 L35 L44 L32 | L41 L38 L44 L35 | L41 L44 L38 | L56 L50 L53 | L53 L59 L50 L56 | L53 L62 L50 L59 | L53 L65 L63 L52 L60 L49 L50 L62 | L53 L52 L63 L65 | L69 L61 A0 L66 L58 | L69 A0 L61 | L64 L69 A0 | A0 L72 L67 L69 L64 | L72 L70 L69 L67 | L22 L27 L25 L24 | A0 L30 L25 L27 L22 | A0 L25 L30 | L33 A0 L25 | L25 L36 L28 A0 L33 | L44 L35 L47 L45 L34 L42 L31 L32 | L32 L31 L42 L44 | L44 L38 L47 L35 | L44 L41 L47 L38 | L44 L47 L41 | L53 L47 L50 | L50 L56 L47 L53 | L50 L59 L47 L56 | L50 L62 L60 L49 L57 L46 L47 L59 | L50 L49 L60 L62 | L66 L58 A0 L63 L55 | L66 A0 L58 | L61 L66 A0 | A0 L69 L64 L66 L61 | L69 L67 L66 L64 | L25 L30 L28 L27 | A0 L33 L28 L30 L25 | A0 L28 L33 | L36 A0 L28 | L28 L39 L31 A0 L36 | L47 L38 L50 L48 L37 L45 L34 L35 | L35 L34 L45 L47 | L47 L41 L50 L38 | L47 L44 L50 L41 | L47 L50 L44 | L47 L53 L44 L50 | L47 L56 L44 L53 | L47 L59 L57 L46 L54 L43 L44 L56 | L47 L46 L57 L59 | L63 L55 A0 L60 L52 | L63 A0 L55 | L58 L63 A0 | A0 L66 L61 L63 L58 | L66 L64 L63 L61 | L28 L33 L31 L30 | A0 L36 L31 L33 L28 | A0 L31 L36 | L39 A0 L31 | L31 L42 L34 A0 L39 | L50 L41 L53 L51 L40 L48 L37 L38 | L38 L37 L48 L50 | L50 L44 L53 L41 | L44 L56 L54 L43 L51 L40 L41 L53 | L44 L43 L54 L56 | L60 L52 A0 L57 L49 | L60 A0 L52 | L55 L60 A0 | A0 L63 L58 L60 L55 | L63 L61 L60 L58 | L31 L36 L34 L33 | A0 L39 L34 L36 L31 | A0 L34 L39 | L42 A0 L34 | L34 L45 L37 A0 L42 | L41 L40 L51 L53 | L57 L49 A0 L54 L46 | L57 A0 L49 | L52 L57 A0 | A0 L60 L55 L57 L52 | L60 L58 L57 L55 | L34 L39 L37 L36 | A0 L42 L37 L39 L34 | A0 L37 L42 | L45 A0 L37 | L37 L48 L40 A0 L45 | L54 L46 A0 L51 L43 | L54 A0 L46 | L49 L54 A0 | A0 L57 L52 L54 L49 | L57 L55 L54 L52 | L37 L42 L40 L39 | A0 L45 L40 L42 L37 | A0 L40 L45 | L48 A0 L40 | L40 L51 L43 A0 L48 | L51 A0 L43 | L46 L51 A0 | A0 L54 L49 L51 L46 | L54 L52 L51 L49 | L40 L45 L43 L42 | A0 L48 L43 L45 L40 | A0 L43 L48 | A0 L51 L46 L48 L43 | L51 L49 L48 L46 | L43 L48 L46 L45
sketch "Sketch5" plane through (0, 0, 13) normal (0, 0, 1) x (1, 0, 0)
  line L0 (-3, 21.8882) -> (3, 21.8882)
  line L1 (3, 21.8882) -> (3, 3)
  line L2 (3, 3) -> (-3, 3)
  line L3 (-3, 3) -> (-3, 21.8882)
  line L4 (-3, 21.8882) -> (3, 3) construction
  line L5 (3, 21.8882) -> (-3, 3) construction
  arc A0 (3, 0) -> (3, 0) centre (0, 0) ccw projected
  point P0 (0, 12.4441)
  dimension "d14" = 6
  constraints: 12 end point, 2 midpoint, 2 parallel, 1 horizontal, 1 perpendicular
  measures "d14" distance of L1.end L2.end
extrude "Extrusion5" cut sketch "Sketch5" against normal blind 6 contours L0 L1 L2 L3
body "Solid1"
